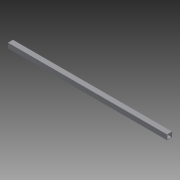
# Autodesk Inventor part: arm-horizontal
Saved by Autodesk Inventor 2014 (Build 180170000, 170)
## iProperties
Created: 2014-03-23
Part Number: arm-horizontal
Material: Generic
Document SubType Name: Modeling
Designer: jferner
Density: 1 g/cm^3
Appearance: Default
Author: jferner
Autodesk Inventor part; units mm, degrees
ref_plane "YZ Plane" through (0, 0, 0) normal (1, 0, 0) x (0, 1, 0)
ref_plane "XZ Plane" through (0, 0, 0) normal (0, 1, 0) x (-1, 0, 0)
ref_plane "XY Plane" through (0, 0, 0) normal (0, 0, 1) x (1, 0, 0)
sketch "Sketch1" plane through (0, 0, 0) normal (1, 0, 0) x (0, 1, 0)
  line L0 (0, 0) -> (19.05, 0)
  line L1 (19.05, 0) -> (19.05, 19.05)
  line L2 (19.05, 19.05) -> (0, 19.05)
  line L3 (0, 19.05) -> (0, 0)
  line L4 (1.5875, 17.4625) -> (17.4625, 17.4625)
  line L5 (17.4625, 17.4625) -> (17.4625, 1.5875)
  line L6 (17.4625, 1.5875) -> (1.5875, 1.5875)
  line L7 (1.5875, 1.5875) -> (1.5875, 17.4625)
  dimension "d0" = 19.05
  dimension "d1" = 19.05
  dimension "d2" = 1.5875
  dimension "d3" = 1.5875
  dimension "d4" = 1.5875
  dimension "d5" = 1.5875
  constraints: 16 end point, 4 parallel, 2 horizontal, 2 perpendicular
  measures "d0" distance of L1.end L2.end
  measures "d1" distance of L0.end L1.end
  measures "d2" distance between parallel lines of L1 L5
  measures "d3" distance between parallel lines of L2 L4
  measures "d4" distance between parallel lines of L3 L7
  measures "d5" distance between parallel lines of L0 L6
extrude "Extrusion1" add sketch "Sketch1" along normal blind 609.6
equation "\"d0\" = sqAlumWidth"
equation "\"d1\" = sqAlumWidth"
equation "\"d2\" = sqAlumWallThickness"
equation "\"d3\" = sqAlumWallThickness"
equation "\"d4\" = sqAlumWallThickness"
equation "\"d5\" = sqAlumWallThickness"
equation "\"sqAlumWidth\" = 19.05"
equation "\"sqAlumWallThickness\" = 1.5875"
body "Solid1"
